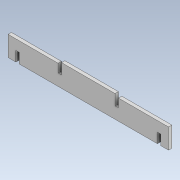
# Autodesk Inventor part: chassis_1_6
Saved by Autodesk Inventor 2022 (Build 260153000, 153)
## iProperties
Created: 2023-04-28
Part Number: chassis_1_6
Material: 一般
Document SubType Name: Modeling
Designer: Johnny Jou
Density: 1 g/cm^3
Appearance: 預設
Author: Johnny Jou
Autodesk Inventor part; units mm, degrees
ref_plane "YZ Plane" through (0, 0, 0) normal (1, 0, 0) x (0, 1, 0)
ref_plane "XZ Plane" through (0, 0, 0) normal (0, 1, 0) x (-1, 0, 0)
ref_plane "XY Plane" through (0, 0, 0) normal (0, 0, 1) x (1, 0, 0)
sketch "草圖1" plane through (0, 0, 0) normal (0, 0, 1) x (1, 0, 0)
  line L0 (0, 0) -> (124, 0)
  line L1 (124, 0) -> (124, -18) construction
  line L2 (124, -18) -> (0, -18)
  line L3 (0, -18) -> (0, 0) construction
  line L4 (35, 0) -> (37.95, 0)
  line L5 (37.95, 0) -> (37.95, -7.5)
  line L6 (37.95, -7.5) -> (35, -7.5)
  line L7 (35, -7.5) -> (35, 0)
  line L8 (89, 0) -> (86.05, 0)
  line L9 (86.05, 0) -> (86.05, -7.5)
  line L10 (86.05, -7.5) -> (89, -7.5)
  line L11 (89, -7.5) -> (89, 0)
  line L12 (134, -18) -> (126.95, -18)
  line L13 (124, 0) -> (134, 0)
  line L14 (134, 0) -> (134, -18)
  line L15 (126.95, -18) -> (126.95, -9)
  line L16 (126.95, -9) -> (124, -9)
  line L17 (0, 0) -> (-10, 0)
  line L18 (-10, 0) -> (-10, -18)
  line L19 (-10, -18) -> (-2.95, -18)
  line L20 (0, -18) -> (0, 0) construction
  line L21 (-2.95, -18) -> (-2.95, -9)
  line L22 (-2.95, -9) -> (0, -9)
  line L23 (0, -9) -> (0, -18)
  line L24 (124, -9) -> (124, -18)
  point P0 (0, -15.5)
  dimension "d0" = 124
  dimension "d1" = 35
  dimension "d3" = 2.95
  dimension "d4" = 2.95
  dimension "d10" = 10.5
  dimension "d16" = 7.5
  dimension "d17" = 35
  dimension "d18" = 2.95
  dimension "d21" = 10
  dimension "d22" = 2.95
  dimension "d23" = 9
  dimension "d24" = 10
  dimension "d25" = 9
  constraints: 50 end point, 10 parallel, 5 horizontal, 5 perpendicular, 4 point on line, 2 collinear
  measures "d0" distance of L1.end L2.end
  measures "d1" distance between parallel lines of L3 L7
  measures "d3" distance of L5.end L6.end
  measures "d4" distance of L9.end L10.end
  measures "d10" distance between parallel lines of L2 L6
  measures "d16" distance of L6.end L4.start
  measures "d17" distance between parallel lines of L1 L11
  measures "d18" distance between parallel lines of L3 L21
  measures "d21" distance between parallel lines of L18 L3
  measures "d22" distance between parallel lines of L1 L15
  measures "d23" distance between parallel lines of L12 L16
  measures "d24" distance between parallel lines of L1 L14
  measures "d25" distance between parallel lines of L19 L22
extrude "擠出1" add sketch "草圖1" along normal blind 3 contours L0 L7 L6 L5 L9 L10 L11 L13 L14 L12 L15 L16 L24 L2 L23 L22 L21 L19 L18 L17
sketch "草圖2" plane through (0, 0, 3) normal (0, 0, 1) x (1, 0, 0)
  line L0 (37.95, 0) -> (86.05, 0)
  line L1 (86.05, 0) -> (86.05, 2)
  line L2 (86.05, 2) -> (37.95, 2)
  line L3 (37.95, 2) -> (37.95, 0)
  line L4 (86.05, -7.5) -> (86.05, 0) projected
  point P0 (0, 0)
  dimension "d26" = 2
  constraints: 8 end point, 2 parallel, 1 collinear, 1 horizontal, 1 perpendicular
  measures "d26" distance between parallel lines of L0 L2
extrude "擠出2" add sketch "草圖2" against normal up to surface (3 mm away)
